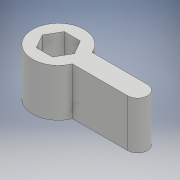
# Autodesk Inventor part: wingnut
Saved by Autodesk Inventor 2018 (Build 220112000, 112)
## iProperties
Created: 2018-11-24
Part Number: wingnut
Material: Generic
Document SubType Name: Modeling
Designer: Prakash
Density: 1 g/cm^3
Appearance: Default
Author: Prakash
Autodesk Inventor part; units mm, degrees
ref_plane "YZ Plane" through (0, 0, 0) normal (1, 0, 0) x (0, 1, 0)
ref_plane "XZ Plane" through (0, 0, 0) normal (0, 1, 0) x (-1, 0, 0)
ref_plane "XY Plane" through (0, 0, 0) normal (0, 0, 1) x (1, 0, 0)
sketch "Sketch1" plane through (0, 0, 0) normal (0, 0, 1) x (1, 0, 0)
  circle A0 centre (0, 0) radius 6.525
  line L0 (-2.0352, -3.525) -> (-4.0703, 0)
  line L1 (-4.0703, 0) -> (-2.0352, 3.525)
  line L2 (-2.0352, 3.525) -> (2.0352, 3.525)
  line L3 (2.0352, 3.525) -> (4.0703, 0)
  line L4 (4.0703, 0) -> (2.0352, -3.525)
  line L5 (2.0352, -3.525) -> (-2.0352, -3.525)
  line L6 (6.0271, 2.5) -> (20, 2.5)
  line L7 (6.0271, -2.5) -> (20, -2.5)
  line L8 (-4.0703, 0) -> (4.0703, 0) construction
  arc A1 (20, -2.5) -> (20, 2.5) centre (20, 0) ccw
  dimension "d0" = 7.05
  dimension "d1" = 3
  dimension "d2" = 5
  dimension "d3" = 20
  constraints: 18 end point, 4 horizontal, 4 point on circle, 2 centre point, 2 coincident, 1 parallel, 1 tangent, 14 other
  measures "d0" distance between parallel lines of L2 L5
  measures "d1" distance edge to line of A0 L2
  measures "d2" distance between parallel lines of L7 L6
  measures "d3" distance of point (0, 0) A1.centre
extrude "Extrusion1" add sketch "Sketch1" along normal blind 12
body "Solid1"
